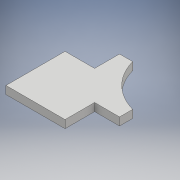
# Autodesk Inventor part: zamek_II_boki
Saved by Autodesk Inventor 2018 (Build 220112000, 112)
## iProperties
Created: 2018-10-22
Part Number: zamek_II_boki
Material: Ogólny
Document SubType Name: Modeling
Designer: EWA
Density: 1 g/cm^3
Appearance: Domyślna
Author: EWA
Autodesk Inventor part; units mm, degrees
ref_plane "YZ Plane" through (0, 0, 0) normal (1, 0, 0) x (0, 1, 0)
ref_plane "XZ Plane" through (0, 0, 0) normal (0, 1, 0) x (-1, 0, 0)
ref_plane "XY Plane" through (0, 0, 0) normal (0, 0, 1) x (1, 0, 0)
sketch "Szkic1" plane through (0, 0, 0) normal (0, 0, 1) x (1, 0, 0)
  line L0 (0, 0) -> (45, 0) construction
  line L1 (45, 0) -> (45, 45) construction
  line L2 (45, 45) -> (0, 45) construction
  line L3 (0, 45) -> (0, 0) construction
  line L4 (0, 45) -> (22.5, 45) construction
  line L5 (45, 0) -> (45, 22.5) construction
  line L6 (22.5, 45) -> (0, 45)
  line L7 (0, 45) -> (0, 0)
  line L8 (0, 0) -> (45, 0)
  line L9 (45, 0) -> (45, 22.5)
  line L10 (22.5, 45) -> (22.5, 64)
  line L11 (45, 22.5) -> (64, 22.5)
  line L12 (22.5, 64) -> (32.5, 64)
  line L13 (64, 22.5) -> (64, 32.5)
  arc A0 (32.5, 64) -> (64, 32.5) centre (75.8985, 75.8985) ccw
  dimension "d0" = 45
  dimension "d1" = 45
  dimension "d2" = 22.5
  dimension "d3" = 19
  dimension "d4" = 19
  dimension "d5" = 10
  dimension "d6" = 10
  dimension "d7" = 45
  constraints: 28 end point, 3 collinear, 3 horizontal, 2 midpoint, 2 parallel, 2 perpendicular, 2 point on circle, 2 vertical, 1 centre point
  measures "d0" distance of L2.end L1.end
  measures "d1" distance of L1.end L0.end
  measures "d2" distance of L2.end L4.end
  measures "d3" distance of L4.end L10.end
  measures "d4" distance of L5.end L11.end
  measures "d5" distance of L10.end L12.end
  measures "d6" distance of L11.end L13.end
  measures "d7" radius of A0
extrude "Wyciągnięcie proste1" add sketch "Szkic1" along normal blind 6
equation "\"d0\" = d1"
equation "\"d3\" = d4"
equation "\"d5\" = d6"
